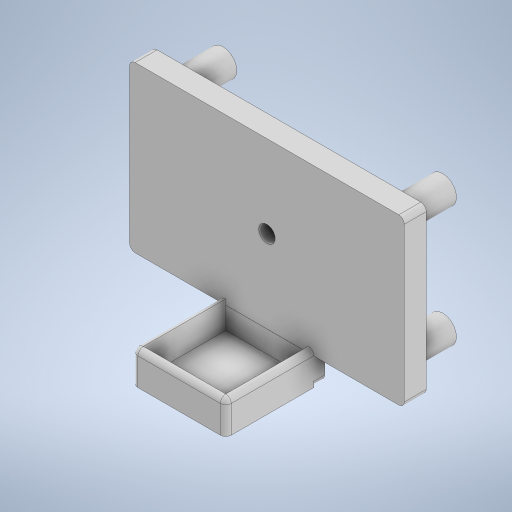
# Autodesk Inventor part: reward v5
Saved by Autodesk Inventor 2023 (Build 270158000, 158)
## iProperties
Created: 2022-07-15
Part Number: reward v5
Material: Generic
Document SubType Name: Modeling
Designer: ledap
Density: 1 g/cm^3
Appearance: Default
Author: ledap
Autodesk Inventor part; units mm, degrees
ref_plane "YZ Plane" through (0, 0, 0) normal (1, 0, 0) x (0, 1, 0)
ref_plane "XZ Plane" through (0, 0, 0) normal (0, 1, 0) x (-1, 0, 0)
ref_plane "XY Plane" through (0, 0, 0) normal (0, 0, 1) x (1, 0, 0)
sketch "Sketch1" plane through (0, 0, 0) normal (0, 0, 1) x (1, 0, 0)
  line L0 (25, 15) -> (-25, 15)
  line L1 (-25, 15) -> (-25, -15)
  line L2 (-25, -15) -> (25, -15)
  line L3 (25, -15) -> (25, 15)
  line L4 (25, 15) -> (-25, -15) construction
  line L5 (-25, 15) -> (25, -15) construction
  point P0 (0, 0)
  dimension "d0" = 50
  dimension "d1" = 30
  constraints: 12 end point, 2 midpoint, 2 parallel, 1 horizontal, 1 perpendicular
  measures "d0" distance of L2.end L1.end
  measures "d1" distance of L1.end L0.end
extrude "Extrusion1" add sketch "Sketch1" along normal blind 4
fillet "Fillet1" radius 1 1 edges at (25, 15, 2)
fillet "Fillet2" radius 1 3 edges at (-25, 15, 2) (25, -15, 2) (-25, -15, 2)
sketch "Sketch4" plane through (0, 0, 4) normal (0, 0, 1) x (1, 0, 0)
  circle A0 centre (0, 0) radius 1.5
  dimension "d19" = 3
  constraints: 1 centre point, 1 coincident
  measures "d19" diameter of A0
hole "Hole2" at (0, 0, 4) direction (0, 0, -1) diameter 3 end through all both
sketch "Sketch6" plane through (0, 0, 4) normal (0, 0, 1) x (1, 0, 0)
  circle A0 centre (-20, 11) radius 2.5
  circle A1 centre (20, 11) radius 2.5
  circle A2 centre (-20, -11) radius 2.5
  circle A3 centre (20, -11) radius 2.5
  line L0 (25, -14) -> (25, 14) projected
  line L1 (-25, 14) -> (-25, -14) projected
  line L2 (24, 15) -> (-24, 15) projected
  line L3 (-24, -15) -> (24, -15) projected
  point P0 (0, 0)
  dimension "d27" = 5
  dimension "d28" = 5
  dimension "d29" = 5
  dimension "d30" = 5
  dimension "d38" = 5
  dimension "d39" = 5
  dimension "d40" = 5
  dimension "d41" = 5
  dimension "d42" = 4
  dimension "d43" = 4
  dimension "d44" = 4
  dimension "d45" = 4
  constraints: 4 centre point
  measures "d27" diameter of A0
  measures "d28" diameter of A1
  measures "d29" diameter of A2
  measures "d30" diameter of A3
  measures "d38" distance from line of L0 A1.centre
  measures "d39" distance from line of L0 A3.centre
  measures "d40" distance from line of L1 A0.centre
  measures "d41" distance from line of L1 A2.centre
  measures "d42" distance from line of A0.centre L2
  measures "d43" distance from line of L2 A1.centre
  measures "d44" distance from line of L3 A2.centre
  measures "d45" distance from line of L3 A3.centre
sketch "Sketch12" plane through (0, 0, 4) normal (0, 0, 1) x (1, 0, 0)
  line L0 (8.5, -20) -> (-8.5, -20)
  line L1 (-8.5, -20) -> (-8.5, -15.0142)
  line L2 (-8.5, -15.0142) -> (8.5, -15.0142)
  line L3 (8.5, -15.0142) -> (8.5, -20)
  line L4 (8.5, -20) -> (-8.5, -15.0142) construction
  line L5 (-8.5, -20) -> (8.5, -15.0142) construction
  line L6 (-24, -15) -> (24, -15) projected
  point P0 (0, 0)
  point P1 (0, -17.5071)
  dimension "d53" = 17
  dimension "d55" = 5
  constraints: 12 end point, 2 midpoint, 2 parallel, 1 horizontal, 1 perpendicular
  measures "d53" distance of L1.end L2.end
  measures "d55" distance between parallel lines of L0 L6
extrude "Extrusion4" add sketch "Sketch12" against normal blind 2
fillet "Fillet3" radius 1 2 edges at (8.5, -20, 3) (-8.5, -20, 3)
sketch "Sketch13" plane through (0, 0, 4) normal (0, 0, 1) x (1, 0, 0)
  line L0 (8.5, -18.9968) -> (-8.5, -18.9968)
  line L1 (-8.5, -18.9968) -> (-8.5, -19.9968)
  line L2 (-8.5, -19.9968) -> (8.5, -19.9968)
  line L3 (8.5, -19.9968) -> (8.5, -18.9968)
  line L4 (8.5, -18.9968) -> (-8.5, -19.9968) construction
  line L5 (-8.5, -18.9968) -> (8.5, -19.9968) construction
  point P0 (0, 0)
  point P1 (0, -19.4968)
  dimension "d59" = 17
  dimension "d60" = 1
  constraints: 12 end point, 2 midpoint, 2 parallel, 1 horizontal, 1 perpendicular
  measures "d59" distance of L2.end L1.end
  measures "d60" distance of L1.end L0.end
extrude "Extrusion5" add sketch "Sketch13" along normal blind 16
sketch "Sketch14" plane through (-8.5, -18.9968, 4) normal (0, 1, 0) x (1, 0, 0)
  line L0 (0, -16) -> (17, -16) projected
  line L1 (0, 0) -> (1, 0)
  line L2 (1, 0) -> (1, -16)
  line L3 (1, -16) -> (0, -16)
  line L4 (0, -16) -> (0, 0)
  point P0 (8.5, 4)
  dimension "d63" = 1
  constraints: 8 end point, 2 parallel, 1 horizontal, 1 perpendicular, 1 point on line
  measures "d63" distance of L2.end L3.end
extrude "Extrusion6" add sketch "Sketch14" along normal blind 5
sketch "Sketch16" plane through (-7.5, -18.9968, 20) normal (0, 1, 0) x (1, 0, 0)
  line L0 (-1, 0) -> (0, 0) projected
  line L1 (0, 0) -> (15, 0)
  line L2 (15, 0) -> (15, 1)
  line L3 (15, 1) -> (0, 1)
  line L4 (0, 1) -> (0, 0)
  point P0 (7.5, 20)
  dimension "d68" = 15
  dimension "d69" = 1
  constraints: 8 end point, 2 parallel, 1 horizontal, 1 perpendicular
  measures "d68" distance of L3.end L2.end
  measures "d69" distance of L2.end L1.end
extrude "Extrusion8" add sketch "Sketch16" along normal blind 5
sketch "Sketch17" plane through (8.5, -18.9968, 20) normal (0, 1, 0) x (1, 0, 0)
  line L0 (0, 16) -> (0, 0) projected
  line L1 (15.5, 16) -> (-32.5, 16) projected
  line L2 (0, 0) -> (-1, 0)
  line L3 (-1, 0) -> (-1, 16)
  line L4 (-1, 16) -> (0, 16)
  line L5 (0, 16) -> (0, 0)
  point P0 (-8.5, 20)
  dimension "d76" = 1
  constraints: 8 end point, 2 parallel, 1 horizontal, 1 perpendicular, 1 point on line
  measures "d76" distance of L3.end L4.end
extrude "Extrusion9" add sketch "Sketch17" along normal blind 5
fillet "Fillet9" radius 1 3 edges at (-8.5, -13.9968, 12) (0, -13.9968, 20) (8.5, -13.9968, 12)
fillet "Fillet10" radius 1 4 edges at (-8.5, -17.4967, 20) (-8.2071, -14.2896, 19.7071) (8.2071, -14.2896, 19.7071) (8.5, -17.4967, 20)
sketch "Sketch18" plane through (0, 0, 0) normal (0, 0, -1) x (-1, 0, 0)
  point P0 (0, 0)
extrude "Extrusion10" add sketch "Sketch6" against normal blind 12
body "Solid1"
